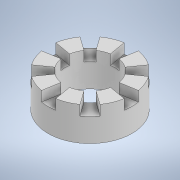
# Autodesk Inventor part: pawn
Saved by Autodesk Inventor 2021.1 (Build 251245010, 245A)
## iProperties
Created: 2021-09-08
Part Number: pawn
Material: Типовые
Document SubType Name: Modeling
Designer: User
Density: 1 g/cm^3
Appearance: По умолчанию
Author: User
Autodesk Inventor part; units mm, degrees
ref_plane "YZ Plane" through (0, 0, 0) normal (1, 0, 0) x (0, 1, 0)
ref_plane "XZ Plane" through (0, 0, 0) normal (0, 1, 0) x (-1, 0, 0)
ref_plane "XY Plane" through (0, 0, 0) normal (0, 0, 1) x (1, 0, 0)
sketch "Эскиз1" plane through (0, 0, 0) normal (0, 1, 0) x (-1, 0, 0)
  circle A0 centre (0, 0) radius 12.5
  circle A1 centre (0, 0) radius 7.5
  dimension "d0" = 25
  dimension "d1" = 15
  constraints: 2 centre point, 2 coincident
  measures "d0" diameter of A0
  measures "d1" diameter of A1
extrude "Выдавливание1" add sketch "Эскиз1" along normal blind 10
sketch "Эскиз2" plane through (0, 10, 0) normal (0, 1, 0) x (1, 0, 0)
  circle A0 centre (0, 0) radius 12.5 projected
  line L0 (-2.1175, 12.3193) -> (0, 0)
  line L1 (2.1175, 12.3193) -> (0, 0)
  line L2 (-10.2084, 7.2138) -> (0, 0)
  line L3 (-7.2138, 10.2084) -> (0, 0)
  line L4 (-12.3193, -2.1175) -> (0, 0)
  line L5 (-12.3193, 2.1175) -> (0, 0)
  line L6 (-7.2138, -10.2084) -> (0, 0)
  line L7 (-10.2084, -7.2138) -> (0, 0)
  line L8 (2.1175, -12.3193) -> (0, 0)
  line L9 (-2.1175, -12.3193) -> (0, 0)
  line L10 (10.2084, -7.2138) -> (0, 0)
  line L11 (7.2138, -10.2084) -> (0, 0)
  line L12 (12.3193, 2.1175) -> (0, 0)
  line L13 (12.3193, -2.1175) -> (0, 0)
  line L14 (7.2138, 10.2084) -> (0, 0)
  line L15 (10.2084, 7.2138) -> (0, 0)
  dimension "d6" = 360
  constraints: 32 end point, 1 coincident, 43 other
extrude "Выдавливание2" cut sketch "Эскиз2" against normal blind 3 contours A0 L13 L12 | L15 L14 A0 | L0 A0 L1 | L2 A0 L3 | L4 A0 L5 | L6 A0 L7 | L8 A0 L9 | L10 A0 L11
